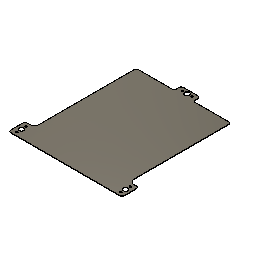
Heated bed (Autodesk Fusion 360 archive; units mm, degrees)
design "Aluminum plate bottom"
Autodesk Fusion 360 part; units mm, degrees
sketch "Sketch1" plane through (0, 0, 0) normal (0, 1, 0) x (1, 0, 0)
  line L0 (0, 0) -> (400, 0)
  line L1 (400, 0) -> (400, 490)
  line L2 (400, 500) -> (250, 500)
  line L3 (0, 490) -> (0, 0)
  line L4 (0, 0) -> (-30, 0)
  line L5 (-40, 10) -> (-40, 60)
  line L6 (-30, 70) -> (-20, 70)
  line L7 (400, 0) -> (430, 0)
  line L8 (440, 10) -> (440, 60)
  line L9 (430, 70) -> (420, 70)
  line L10 (240, 510) -> (240, 520)
  line L11 (160, 520) -> (160, 510)
  arc A0 (-30, 70) -> (-40, 60) centre (-30, 60) ccw
  arc A1 (-40, 10) -> (-30, 0) centre (-30, 10) ccw
  arc A2 (440, 60) -> (430, 70) centre (430, 60) ccw
  arc A3 (430, 0) -> (440, 10) centre (430, 10) ccw
  line L12 (375, 25) -> (375, 475) construction
  line L13 (375, 475) -> (25, 475) construction
  line L14 (25, 475) -> (25, 25) construction
  line L15 (25, 25) -> (375, 25) construction
  arc A4 (400, 90) -> (420, 70) centre (420, 90) ccw
  arc A5 (-20, 70) -> (0, 90) centre (-20, 90) ccw
  line L16 (-25, 70) -> (-20, 70)
  line L17 (-20, 0) -> (-25, 0)
  line L18 (170, 530) -> (230, 530)
  arc A6 (170, 530) -> (160, 520) centre (170, 520) ccw
  arc A7 (240, 520) -> (230, 530) centre (230, 520) ccw
  arc A8 (240, 510) -> (250, 500) centre (250, 510) ccw
  line L19 (0, 500) -> (150, 500)
  arc A9 (150, 500) -> (160, 510) centre (150, 510) ccw
  line L20 (10, 500) -> (390, 500) construction
  line L21 (200, 530) -> (200, 500) construction
  arc A10 (10, 500) -> (0, 490) centre (10, 490) ccw
  arc A11 (400, 490) -> (390, 500) centre (390, 490) ccw
  line L22 (180, 515) -> (220, 515) construction
  circle A12 centre (220, 515) radius 4
  circle A13 centre (200, 515) radius 10
  circle A14 centre (180, 515) radius 4
  line L23 (440, 35) -> (400, 35) construction
  line L24 (420, 35) -> (420, 55) construction
  line L25 (420, 35) -> (420, 15) construction
  circle A15 centre (420, 35) radius 10
  circle A16 centre (420, 55) radius 4
  circle A17 centre (420, 15) radius 4
  line L26 (-40, 35) -> (0, 35) construction
  line L27 (-20, 35) -> (-20, 15) construction
  line L28 (-20, 35) -> (-20, 55) construction
  circle A18 centre (-20, 35) radius 10
  circle A19 centre (-20, 15) radius 4
  circle A20 centre (-20, 55) radius 4
  point P0 (-40, 0)
  point P1 (-40, 70)
  point P2 (440, 0)
  point P3 (440, 70)
  point P4 (240, 530)
  point P5 (160, 530)
  dimension "d1" = 500
  dimension "d2" = 400
  dimension "d4" = 70
  dimension "d6" = 70
  dimension "d7" = 80
  dimension "d12" = 10
  dimension "d13" = 20
  dimension "d14" = 10
  dimension "d15" = 10
  dimension "d16" = 30
  dimension "d17" = 10
  dimension "d18" = 200
  dimension "d19" = 20
  dimension "d20" = 8
  dimension "d21" = 8
  dimension "d22" = 20
  dimension "d23" = 20
  dimension "d26" = 20
  dimension "d27" = 20
  dimension "d28" = 20
  dimension "d29" = 8
  dimension "d30" = 8
  dimension "d35" = 40
  dimension "d36" = 40
  dimension "d37" = 20
  dimension "d38" = 20
  dimension "d39" = 20
  dimension "d40" = 8
  dimension "d41" = 8
  measures "d1" distance of L0.start L19.start
  measures "d2" distance of L0.start L0.end
  measures "d4" distance of P0 P1
  measures "d6" distance of P2 P3
  measures "d7" distance of P4 P5
  measures "d12" radius of A0
  measures "d13" radius of A4
  measures "d14" radius of A6
  measures "d15" radius of A9
  measures "d16" distance of L2 L18
  measures "d17" radius of A10
  measures "d18" distance of L3 L21
  measures "d19" diameter of A13
  measures "d20" diameter of A12
  measures "d21" diameter of A14
  measures "d22" distance of A13.centre L22.start
  measures "d23" distance of L22.end A13.centre
  measures "d26" diameter of A15
  measures "d27" distance of L24.end L24.start
  measures "d28" distance of L25.end L24.start
  measures "d29" diameter of A16
  measures "d30" diameter of A17
  measures "d35" distance of L1 L8
  measures "d36" distance of L3 L5
  measures "d37" distance of L27.start L28.end
  measures "d38" distance of L27.start L27.end
  measures "d39" diameter of A18
  measures "d40" diameter of A19
  measures "d41" diameter of A20
extrude "Extrude5" add sketch "Sketch1" along normal blind 2
extrude "Extrude1" [suppressed]
extrude "Extrude2" [suppressed]
extrude "Extrude3" [suppressed]
extrude "Extrude4" [suppressed]
equation "d18 = d2 / 2"

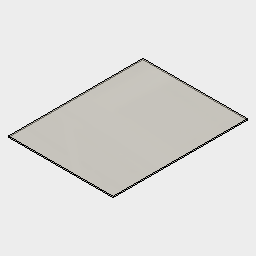
design "Glass top"
Autodesk Fusion 360 part; units mm, degrees
sketch "Sketch1" plane through (0, 0, 0) normal (0, 1, 0) x (1, 0, 0)
  line L0 (0, 0) -> (350, 0)
  line L1 (350, 0) -> (350, -450)
  line L2 (350, -450) -> (0, -450)
  line L3 (0, -450) -> (0, 0)
  dimension "d1" = 350
  dimension "d2" = 450
  measures "d1" distance of L0.start L0.end
  measures "d2" distance of L3.end L2.end L0
extrude "Extrude1" add sketch "Sketch1" along normal blind 4

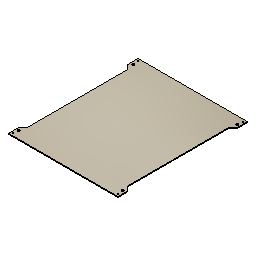
design "Aluminum plate between silicon and groundplane"
Autodesk Fusion 360 part; units mm, degrees
sketch "Sketch1" plane through (0, 0, 0) normal (0, 1, 0) x (1, 0, 0)
  line L0 (0, 0) -> (350, 0)
  line L1 (350, 0) -> (350, 450)
  line L2 (350, 450) -> (0, 450)
  line L3 (0, 450) -> (0, 0)
  line L4 (0, 0) -> (-15, 0)
  line L5 (-15, 0) -> (-15, 35)
  line L6 (-15, 35) -> (0, 35)
  line L7 (0, 35) -> (0, 0)
  line L8 (350, 0) -> (365, 0)
  line L9 (365, 0) -> (365, 35)
  line L10 (365, 35) -> (350, 35)
  line L11 (350, 35) -> (350, 0)
  line L12 (162.5, 450) -> (187.5, 450)
  line L13 (350, 450) -> (365, 450)
  line L14 (365, 450) -> (365, 415)
  line L15 (365, 415) -> (350, 415)
  line L16 (350, 415) -> (350, 450)
  line L17 (0, 450) -> (-15, 450)
  line L18 (-15, 450) -> (-15, 415)
  line L19 (-15, 415) -> (0, 415)
  line L20 (0, 415) -> (0, 450)
  line L21 (-15, 415) -> (0, 400)
  line L22 (365, 415) -> (350, 400)
  line L23 (365, 35) -> (350, 50)
  line L24 (-15, 35) -> (0, 50)
  circle A0 centre (-7.5, 442) radius 2.5
  circle A1 centre (-5.5, 424) radius 4
  line L25 (175, 0) -> (175, 450) construction
  line L26 (350, 225) -> (0, 225) construction
  circle A2 centre (-5.5, 26) radius 4
  circle A3 centre (-7.5, 8) radius 2.5
  circle A4 centre (355.5, 26) radius 4
  circle A5 centre (357.5, 8) radius 2.5
  circle A6 centre (357.5, 442) radius 2.5
  circle A7 centre (355.5, 424) radius 4
  line L27 (-7.5, 442) -> (-7.5, 450) construction
  dimension "d1" = 450
  dimension "d2" = 350
  dimension "d3" = 15
  dimension "d4" = 35
  dimension "d5" = 15
  dimension "d6" = 35
  dimension "d11" = 35
  dimension "d12" = 15
  dimension "d13" = 15
  dimension "d14" = 15
  dimension "d15" = 15
  dimension "d16" = 5
  dimension "d17" = 8
  dimension "d18" = 8
  dimension "d22" = 0
  dimension "d23" = 0
  dimension "d24" = 9
  dimension "d25" = 2
  constraint horizontal L0
  constraint vertical L1
  constraint horizontal L2
  constraint vertical L3
  constraint coincident L0.start L3.end
  constraint horizontal L4
  constraint vertical L5
  constraint horizontal L6
  constraint vertical L7
  constraint horizontal L8
  constraint vertical L9
  constraint horizontal L10
  constraint vertical L11
  constraint horizontal L12
  constraint coincident L2 L12.start
  constraint horizontal L13
  constraint vertical L14
  constraint horizontal L15
  constraint vertical L16
  constraint horizontal L17
  constraint vertical L18
  constraint horizontal L19
  constraint vertical L20
  constraint collinear L9 L14
  constraint collinear L5 L18
  constraint collinear L15 L19
  constraint coincident L3 L21.end
  constraint coincident L1 L22.end
  constraint coincident L1 L23.end
  constraint coincident L3 L24.end
  constraint midpoint L0 L25.start
  constraint midpoint L12 L25.end
  constraint perpendicular L12 L25
  constraint midpoint L1 L26.start
  constraint midpoint L3 L26.end
  constraint symmetric A0 L26 A3
  constraint symmetric A1 L26 A2
  constraint symmetric A0 L25 A6
  constraint symmetric A1 L25 A7
  constraint symmetric L25 A2 A4
  constraint symmetric L25 A3 A5
  constraint coincident A0.centre L27.start
  constraint midpoint L17 L27.end
  constraint perpendicular L17 L27
  measures "d1" vertical distance of L0.start L2.end
  measures "d2" horizontal distance of L0.start L0.end
  measures "d3" horizontal distance of L5.end L6.end
  measures "d4" vertical distance of L4.end L5.end
  measures "d5" horizontal distance of L9.end L10.end
  measures "d6" vertical distance of L8.end L9.end
  measures "d11" distance of L13.end L14.end
  measures "d12" distance of L19.end L21.end
  measures "d13" distance of L6.end L24.end
  measures "d14" vertical distance of L9.end L23.end
  measures "d15" vertical distance of L14.end L22.end
  measures "d16" diameter of A0
  measures "d17" diameter of A1
  measures "d18" vertical distance of L17.end A0.centre
  measures "d24" vertical distance of L18.end A1.centre
  measures "d25" horizontal distance of A0.centre A1.centre
extrude "Extrude1" add sketch "Sketch1" along normal blind 3
equation "d3 = d5"
equation "d4 = d6"
equation "d11 = d6"
equation "d12 = d5"
equation "d13 = d5"
equation "d14 = d5"
equation "d15 = d14"
